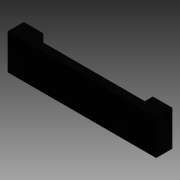
# Autodesk Inventor part: FlatFlex26
Saved by Autodesk Inventor 2014 (Build 180170000, 170)
## iProperties
Created: 2015-03-25
Part Number: FlatFlex26
Material: Generic
Document SubType Name: Modeling
Designer: Owner
Density: 1 g/cm^3
Appearance: Black
Author: Owner
Autodesk Inventor part; units mm, degrees
ref_plane "YZ Plane" through (0, 0, 0) normal (1, 0, 0) x (0, 1, 0)
ref_plane "XZ Plane" through (0, 0, 0) normal (0, 1, 0) x (-1, 0, 0)
ref_plane "XY Plane" through (0, 0, 0) normal (0, 0, 1) x (1, 0, 0)
sketch "Sketch1" plane through (0, 0, 0) normal (0, 0, 1) x (1, 0, 0)
  line L0 (8.0225, -1.3281) -> (-10.4075, -1.3281)
  line L1 (-10.4075, -1.3281) -> (-10.4075, 3.0719)
  line L2 (-10.4075, 3.0719) -> (8.0225, 3.0719)
  line L3 (8.0225, 3.0719) -> (8.0225, -1.3281)
  point P0 (0, 0)
  dimension "d0" = 18.43
  dimension "d1" = 4.4
  constraints: 8 end point, 2 parallel, 1 horizontal, 1 perpendicular
  measures "d0" distance of L1.end L2.end
  measures "d1" distance of L2.end L0.start
extrude "Extrusion1" add sketch "Sketch1" along normal blind 2
sketch "Sketch2" plane through (-10.4075, 3.0719, 0) normal (0, 1, 0) x (1, 0, 0)
  line L0 (0, 0) -> (18.43, 0) projected
  line L1 (18.43, 0) -> (18.43, -2) projected
  line L2 (2.415, 0) -> (16.015, 0)
  line L3 (16.015, 0) -> (16.015, -1)
  line L4 (16.015, -1) -> (2.415, -1)
  line L5 (2.415, -1) -> (2.415, 0)
  point P0 (10.4075, 0)
  dimension "d4" = 13.6
  dimension "d5" = 2.415
  dimension "d6" = 0
  dimension "d7" = 1
  constraints: 8 end point, 2 parallel, 1 horizontal, 1 perpendicular
  measures "d4" distance of L2.start L2.end
  measures "d5" distance between parallel lines of L1 L3
  measures "d6" distance between parallel lines of L0 L2
  measures "d7" distance of L2.end L3.end
extrude "Extrusion2" cut sketch "Sketch2" against normal blind 1
body "Solid1"
